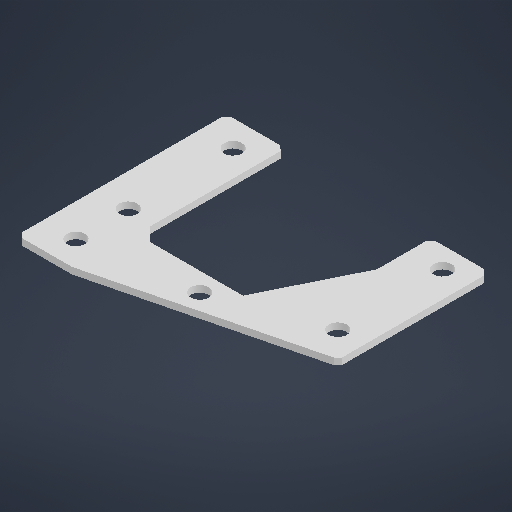
# Autodesk Inventor part: backFunnel
Saved by Autodesk Inventor 2025.2 (Build 292293000, 293)
## iProperties
Created: 2025-03-23
Part Number: backFunnel
Material: Generic
Document SubType Name: Modeling
Designer: Jahan
Density: 1 g/cm^3
Appearance: Default
Author: Jahan
Autodesk Inventor part; units mm, degrees
ref_plane "YZ Plane" through (0, 0, 0) normal (1, 0, 0) x (0, 1, 0)
ref_plane "XZ Plane" through (0, 0, 0) normal (0, 1, 0) x (-1, 0, 0)
ref_plane "XY Plane" through (0, 0, 0) normal (0, 0, 1) x (1, 0, 0)
sketch "Sketch1" plane through (0, 0, 0) normal (0, 1, 0) x (-1, 0, 0)
  circle A0 centre (28.5676, 25.8614) radius 2.1844
  circle A1 centre (28.5676, -12.2386) radius 2.1844
  circle A2 centre (28.5676, 13.1614) radius 2.1844
  circle A3 centre (-22.2324, -12.2386) radius 2.1844
  circle A4 centre (-22.2324, 13.1614) radius 2.1844
  line L0 (23.2336, 32.2114) -> (-27.5664, 19.5114)
  line L1 (-27.5664, 19.5114) -> (-28.5824, 18.4954)
  line L2 (23.2336, 32.2114) -> (34.1239, 32.2114)
  line L3 (35.2397, -18.5886) -> (23.4876, -18.5886)
  line L4 (36.5097, 30.9154) -> (36.5097, -17.3186)
  line L5 (22.2214, 14.3333) -> (22.2214, -17.4167)
  line L6 (19.0464, 17.5083) -> (-2.1664, 17.5083)
  line L7 (-14.2949, -16.0486) -> (-15.5649, -17.3186)
  line L8 (-27.3124, -17.3186) -> (-28.5824, -16.0486)
  line L9 (22.2214, 14.3333) -> (19.0464, 17.5083)
  line L10 (36.5097, 30.9154) -> (35.24, 32.2114)
  line L11 (36.5097, -17.3186) -> (35.2397, -18.5886)
  line L12 (23.4876, -18.5886) -> (22.2214, -17.4167)
  line L13 (35.24, 32.2114) -> (34.1239, 32.2114)
  line L14 (-15.5649, -17.3186) -> (-27.3124, -17.3186)
  line L15 (-28.5824, -16.0486) -> (-28.5824, 18.4954)
  line L16 (-14.2949, -12.2386) -> (-14.2949, -16.0486)
  line L17 (-14.2949, -12.2386) -> (-14.2949, -4.3011)
  line L18 (-3.5693, 17.5083) -> (-14.2949, -4.3011)
  line L19 (-2.1664, 17.5083) -> (-3.5693, 17.5083)
  circle A5 centre (2.3498, 22.0704) radius 2.1844
  point P0 (0, 0)
  point P1 (36.5051, 32.2114)
  dimension "d0" = 31.75
  dimension "d6" = 4.3688
  constraints: 40 end point, 6 centre point, 5 horizontal, 4 vertical, 1 parallel, 1 perpendicular
  measures "d0" distance of L9.start L5.end
  measures "d6" diameter of A5
extrude "Extrusion1" add sketch "Sketch1" along normal blind 1.5875
body "Solid1"
